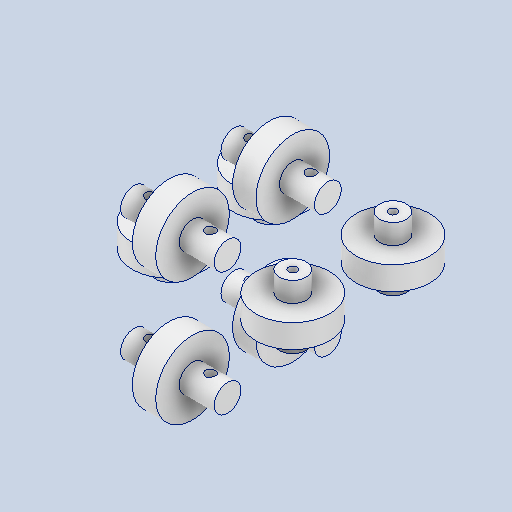
# Autodesk Inventor part: belt_liner_v2_B_unit
Saved by Autodesk Inventor 2025.2 (Build 292293000, 293)
## iProperties
Created: 2025-01-05
Part Number: belt_liner_v2_B_unit
Material: アルミニウム 6061
Document SubType Name: Modeling
Designer: haruy
Density: 2.7 g/cm^3
Appearance: アルミニウム - フラット
Author: haruy
Autodesk Inventor part; units mm, degrees
ref_plane "YZ Plane" through (0, 0, 0) normal (1, 0, 0) x (0, 1, 0)
ref_plane "XZ Plane" through (0, 0, 0) normal (0, 1, 0) x (-1, 0, 0)
ref_plane "XY Plane" through (0, 0, 0) normal (0, 0, 1) x (1, 0, 0)
derived "belt_liner_v2_Sketch_Base.ipt"
ref_plane "作業平面2" through (0, 281.5, 0) normal (0, 1, 0) x (-1, 0, 0)
sketch "スケッチ4" plane through (0, 300, 0) normal (0, 1, 0) x (-1, 0, 0)
  line L0 (0, 0) -> (-15, 0) projected
  line L1 (-15, 0) -> (-15, -578.917) projected
  line L2 (-15, -578.917) -> (0, -578.917) projected
  line L3 (0, -578.917) -> (0, 0) projected
  line L4 (-4, -22.5) -> (-11, -22.5) projected
  line L5 (-11, -22.5) -> (-11, -0.5) projected
  line L6 (-11, -0.5) -> (-4, -0.5) projected
  line L7 (-4, -0.5) -> (-4, -22.5) projected
  line L8 (-4, -11.5) -> (-11, -11.5) projected
  line L9 (-4, -30.5) -> (-11, -30.5) projected
  line L10 (-11, -30.5) -> (-11, -52.5) projected
  line L11 (-11, -52.5) -> (-4, -52.5) projected
  line L12 (-4, -52.5) -> (-4, -30.5) projected
  line L13 (-4, -41.5) -> (-11, -41.5) projected
  line L14 (6.5, -7.5) -> (-21.5, -7.5) projected
  line L15 (-21.5, -7.5) -> (-21.5, -15.5) projected
  line L16 (-21.5, -15.5) -> (6.5, -15.5) projected
  line L17 (6.5, -15.5) -> (6.5, -7.5) projected
  line L18 (-11.5, -23) -> (-3.5, -23) projected
  line L19 (-3.5, -23) -> (-3.5, 0) projected
  line L20 (-3.5, 0) -> (-11.5, 0) projected
  line L21 (-11.5, 0) -> (-11.5, -23) projected
  circle A0 centre (1.5, -11.5) radius 4 projected
  circle A1 centre (-16.5, -11.5) radius 4 projected
  circle A2 centre (-26, -26.5) radius 11 projected
  circle A3 centre (-26, -26.5) radius 4 projected
  line L22 (-7.5, -52.5) -> (-7.5, 0) projected
  line L23 (0, -26.5) -> (-15, -26.5) projected
  circle A4 centre (11, -26.5) radius 11 projected
  circle A5 centre (11, -26.5) radius 4 projected
  circle A6 centre (1.5, -41.5) radius 4 projected
  line L24 (6.5, -37.5) -> (6.5, -45.5) projected
  line L25 (6.5, -45.5) -> (-21.5, -45.5) projected
  line L26 (-21.5, -45.5) -> (-21.5, -37.5) projected
  circle A7 centre (-16.5, -41.5) radius 4 projected
  line L27 (-21.5, -37.5) -> (6.5, -37.5) projected
  circle A8 centre (11, -56.5) radius 11 projected
  circle A9 centre (11, -56.5) radius 4 projected
  circle A10 centre (-26, -56.5) radius 11 projected
  circle A11 centre (-26, -56.5) radius 4 projected
  circle A12 centre (11, -56.5) radius 1.5 projected
  circle A13 centre (1.5, -41.5) radius 1.25 projected
  circle A14 centre (-16.5, -41.5) radius 1.25 projected
  circle A15 centre (-26, -56.5) radius 1.5 projected
  circle A16 centre (11, -26.5) radius 1.5 projected
  circle A17 centre (-26, -26.5) radius 1.5 projected
  circle A18 centre (1.5, -11.5) radius 1.25 projected
  circle A19 centre (-16.5, -11.5) radius 1.25 projected
  line L28 (22, 0) -> (-37, 0) projected
  line L29 (-37, 0) -> (-37, -67.5) projected
  line L30 (-37, -67.5) -> (22, -67.5) projected
  line L31 (22, -67.5) -> (22, 0) projected
  line L32 (-23, 0) -> (-28, 0) projected
  line L33 (-28, 0) -> (-28, -41) projected
  line L34 (-28, -41) -> (-23, -41) projected
  line L35 (-23, -41) -> (-23, 0) projected
  line L36 (-23, -10) -> (-28, -10) projected
  circle A20 centre (-25.5, -16) radius 1.25 projected
  circle A21 centre (-25.5, -16) radius 4 projected
  circle A22 centre (-25.5, -36) radius 4 projected
  circle A23 centre (-25.5, -36) radius 1.25 projected
  circle A24 centre (10.5, -36) radius 1.25 projected
  circle A25 centre (10.5, -16) radius 1.25 projected
  line L37 (6.5, -11.5) -> (-21.5, -11.5)
  line L38 (6.5, -41.5) -> (-21.5, -41.5)
  line L39 (2, 16.7328) -> (-17, 16.7328) projected
  line L40 (-17, 16.7328) -> (-17, 66.7328) projected
  line L41 (-17, 66.7328) -> (2, 66.7328) projected
  line L42 (2, 66.7328) -> (2, 16.7328) projected
  line L43 (-17, 61.7819) -> (-23, 61.7819) projected
  line L44 (-23, 61.7819) -> (-23, 36.7819) projected
  line L45 (-23, 36.7819) -> (-17, 36.7819) projected
  line L46 (-17, 36.7819) -> (-17, 61.7819) projected
  line L47 (18, 61.7819) -> (-33, 61.7819) projected
  line L48 (-33, 61.7819) -> (-33, 27.0059) projected
  line L49 (-33, 27.0059) -> (18, 27.0059) projected
  line L50 (18, 27.0059) -> (18, 61.7819) projected
  line L51 (-1.15, 66.7328) -> (-13.85, 66.7328) projected
  line L52 (-13.85, 66.7328) -> (-13.85, 140.5976) projected
  line L53 (-13.85, 140.5976) -> (-1.15, 140.5976) projected
  line L54 (-1.15, 140.5976) -> (-1.15, 66.7328) projected
  line L55 (7.85, 70.1693) -> (-22.85, 70.1693) projected
  line L56 (-22.85, 70.1693) -> (-22.85, 74.1693) projected
  line L57 (-22.85, 74.1693) -> (7.85, 74.1693) projected
  line L58 (7.85, 74.1693) -> (7.85, 70.1693) projected
  circle A26 centre (-17.85, 72.1693) radius 4 projected
  point P0 (-7.5, 0)
  point P1 (-4, -15.5)
  point P2 (-11, -15.5)
  point P3 (-4, -45.5)
  point P4 (-11, -45.5)
  point P5 (-7.5, 0)
  constraints: 4 end point, 4 midpoint
extrude "押し出し1" add sketch "スケッチ4" along normal mid plane 7 from surface at -18.5 contours A4 A25 | A25 A4 | A8 | A2 A22 L35 A3 A21 | A21 L35 A2 | A2 L35 A22 | L35 A21 L33 A2 A20 | L35 A3 L33 A21 | A2 L33 A22 L35 | A10 | A2 A21 L33 A3 A22 | A20 A2 | A21 A2 L33 | A2 A22 L33 | A22 L33 A3 L35 | A23 | A24 picked at (7.6811, -33.5053) picked at (10.5247, -16.0944) picked at (-22.8135, -17.8721) picked at (-22.7897, -34.4904) picked at (-27.5222, -17.1525) picked at (-27.5712, -35.2983) picked at (-25.5178, -16.095) picked at (-28.2066, -17.7697) picked at (-28.2137, -34.5725)
ref_plane "作業平面4" through (0, 291, 0) normal (0, 1, 0) x (-1, 0, 0)
extrude "押し出し2" add sketch "スケッチ4" along normal mid plane 19 from surface at -18.5 separate body contours L35 A3 L33 | A3 L35 | L33 A3 | A5 | A9 | A11 | A12 | A15 | A16 | A17
revolve "回転1" add sketch "スケッチ4" angle 360 about axis through (-6.5, 300, -11.5) along (1, 0, 0) separate body picked at (4.5499, -11.2033) picked at (-0.2765, -9.1801) picked at (1.5502, -11.0864) picked at (-14.7235, -9.1801) picked at (-19.5499, -11.2033) picked at (-16.4498, -11.0864) contours L14 A0 L3 | L3 A0 L37 L19 L14 | L19 L37 L7 L14 | A0 L37 A18 L3 | L3 L37 A0 | L14 L17 L37 A0 | L7 L8 L22 L14 | L21 L37 A1 L1 L14 | L14 L5 L37 L21 | L22 L8 L5 L14 | A18 L37 | L1 A1 L14 | A1 L37 L1 | L1 L37 A19 A1 | A1 L37 L15 L14 | L37 A19
revolve "回転2" add sketch "スケッチ4" angle 360 about axis through (4, 300, -41.5) along (1, 0, 0) separate body picked at (4.5499, -41.7967) picked at (-0.2765, -43.8199) picked at (1.8294, -42.2189) picked at (-14.7235, -43.8199) picked at (-19.5499, -41.7967) picked at (-16.0833, -41.8873) contours L25 L12 L38 A6 L3 | L3 A6 L25 | L38 A13 A6 L3 | L3 A6 L38 | L12 L25 L22 L13 | L38 L24 L25 A6 | L38 A13 | L22 L25 L10 L13 | L10 L25 L1 A7 L38 | L38 A7 L1 | L1 A7 L38 A14 | A7 L25 L26 L38 | L25 A7 L1 | A14 L38
revolve "回転3" add sketch "スケッチ4" angle 360 about axis through (-6.5, 300, -11.5) along (1, 0, 0) separate body contours L7 L4 L22 L16 | L22 L4 L5 L16
revolve "回転4" add sketch "スケッチ4" angle 360 about axis through (-6.5, 300, -41.5) along (1, 0, 0) separate body contours L12 L11 L22 L25 | L22 L11 L10 L25
sketch "スケッチ2" plane through (-11, 291, -26.5) normal (0, 1, 0) x (1, 0, 0)
  circle A0 centre (0, 0) radius 4 projected
  circle A1 centre (0, 0) radius 1.25
  circle A2 centre (37, 0) radius 4 projected
  circle A3 centre (37, 0) radius 1.25
  circle A4 centre (0, 30) radius 4 projected
  circle A5 centre (0, 30) radius 1.25
  circle A6 centre (37, 30) radius 4 projected
  circle A7 centre (37, 30) radius 1.25
  point P0 (11, -26.5)
  dimension "d11" = 2.5
  dimension "d12" = 2.5
  dimension "d13" = 2.5
  dimension "d14" = 2.5
  constraints: 4 centre point, 4 coincident
  measures "d11" diameter of A1
  measures "d12" diameter of A3
  measures "d13" diameter of A5
  measures "d14" diameter of A7
extrude "押し出し3" cut sketch "スケッチ2" against normal blind 5 contours A1 | A3 | A5 | A7 bodies 2
ref_plane "作業平面5" through (7.5, 304, -11.5) normal (0, 1, 0) x (-1, 0, 0)
sketch "スケッチ3" plane through (7.5, 304, -11.5) normal (0, 1, 0) x (-1, 0, 0)
  line L0 (14, -26) -> (14, -34) projected
  line L1 (14, 4) -> (14, -4) projected
  line L2 (-14, -26) -> (-14, -34) projected
  line L3 (-14, 4) -> (-14, -4) projected
  point P0 (7.5, 11.5)
  point P1 (9, 0)
  point P2 (-9, 0)
  point P3 (9, -30)
  point P4 (-9, -30)
  dimension "d17" = 5
  dimension "d18" = 5
  dimension "d19" = 5
  dimension "d20" = 5
  measures "d17" distance from line of point (9, -30) L0
  measures "d18" distance from line of L1 point (9, 0)
  measures "d19" distance from line of point (-9, -30) L2
  measures "d20" distance from line of point (-9, 0) L3
hole "穴1" at (-1.5, 304, -11.5) at (16.5, 304, -11.5) at (16.5, 304, -41.5) at (-1.5, 304, -41.5) direction (0, -1, 0) diameter 3 end through all bodies 3 4
mirror "ミラー1" about plane through (0, 281.5, 0) normal (0, 1, 0) bodies 3 5 4 6
mirror "ミラー2" about plane through (0, 281.5, 0) normal (0, 1, 0) of "押し出し3" bodies 2
ref_plane "作業平面3" through (0, 300, 0) normal (0, 1, 0) x (-1, 0, 0)
equation "\"d18\" = d17"
equation "\"d19\" = d17"
equation "\"d20\" = d17"
